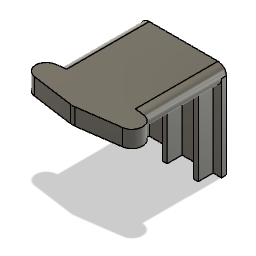
ServoBarMount (Autodesk Fusion 360 design; units mm, degrees)
Autodesk Fusion 360 part; units mm, degrees
sketch "Sketch1" plane through (0, 0, 0) normal (0, 1, 0) x (1, 0, 0)
  line L0 (0, 0) -> (16.3, 0) construction
  line L1 (2.9047, 2.75) -> (2.9047, -2.75) construction
  line L2 (2.9047, 2.75) -> (14.4306, 1.9957)
  line L3 (2.9047, -2.75) -> (14.4306, -1.9957)
  line L4 (0, 4) -> (0, -4) construction
  arc A0 (14.4306, -1.9957) -> (14.4306, 1.9957) centre (14.3, 0) ccw
  line L5 (0.7832, 5.545) -> (14.8035, 3.5646)
  line L6 (0.7832, -5.545) -> (14.8035, -3.5646)
  arc A1 (14.8035, -3.5646) -> (14.8035, 3.5646) centre (14.3, 0) ccw
  line L7 (-2.9047, 2.75) -> (-14.4306, 1.9957)
  line L8 (-0.7832, 5.545) -> (-14.8035, 3.5646)
  line L9 (-2.9047, -2.75) -> (-14.4306, -1.9957)
  line L10 (-0.7832, -5.545) -> (-14.8035, -3.5646)
  arc A2 (-14.4306, 1.9957) -> (-14.4306, -1.9957) centre (-14.3, 0) ccw
  arc A3 (-14.8035, 3.5646) -> (-14.8035, -3.5646) centre (-14.3, 0) ccw
  arc A4 (0.7832, 5.545) -> (-0.7832, 5.545) centre (0, 0) ccw
  arc A5 (-0.7832, -5.545) -> (0.7832, -5.545) centre (0, 0) ccw
  arc A6 (2.9047, 2.75) -> (-2.9047, 2.75) centre (0, 0) ccw
  arc A7 (-2.9047, -2.75) -> (2.9047, -2.75) centre (0, 0) ccw
  line L11 (14.3, 3.6357) -> (14.3, 31.6)
  line L12 (14.3, 30) -> (-14.3, 30)
  line L13 (-14.3, 30) -> (-14.3, 3.6357)
  line L14 (14.3, 31.6) -> (-14.3, 31.6)
  line L15 (-14.3, 31.6) -> (-14.3, 30)
  dimension "d1" = 8
  dimension "d2" = 16.3
  dimension "d3" = 4
  dimension "d5" = 5.5
  dimension "d6" = 1.6
  dimension "d7" = 1.6
  dimension "d8" = 30
  dimension "d16" = 1.6
  constraint coincident L0.start A4.centre
  constraint horizontal L0
  constraint coincident L0 A0.centre
  constraint coincident L0.end A0
  constraint vertical L1
  constraint tangent L2 A0
  constraint tangent L3 A0
  constraint coincident L4.start A6
  constraint coincident L4.end A6
  constraint perpendicular L0 L4
  constraint concentric A0 A1
  constraint concentric A4 A6
  constraint tangent L5 A1
  constraint tangent L5 A4
  constraint tangent L6 A1
  constraint tangent L6 A4
  constraint symmetric L1.start L4 L7.start
  constraint symmetric L1.end L4 L9.start
  constraint symmetric L2.end L4 L7.end
  constraint symmetric L3.end L4 L9.end
  constraint symmetric L4 A0 A2
  constraint symmetric L4 L5.start L8.start
  constraint symmetric L4 L5.end L8.end
  constraint symmetric L4 L6.start L10.start
  constraint symmetric L4 L6.end L10.end
  constraint symmetric L4 A1 A3
  constraint coincident L9.start A6
  constraint concentric A4 A5
  constraint tangent L10 A5
  constraint concentric A6 A7
  constraint vertical L11
  constraint horizontal L12
  constraint vertical L13
  constraint coincident L8 L13.end
  constraint vertical A0.centre L11.start
  constraint vertical A2.centre L13.end
  constraint coincident L5 L11.start
  constraint horizontal L14
  constraint vertical L15
  constraint coincident L11.end L14.start
  constraint coincident L12.start L11
  measures "d1" diameter of A6
  measures "d2" distance of L0.start L0.end
  measures "d3" diameter of A0
  measures "d5" distance of L1.start L1.end
  measures "d6" distance of A0 A1
  measures "d7" distance of A4 A6
  measures "d8" distance of L0.start L12
  measures "d16" distance of L12.end L14.end
extrude "Extrude1" add sketch "Sketch1" along normal blind 1.6 contours L2 L3 A0 L7 L9 A2 A6 A7 | L5 L8 A4 L11 L12 L13 | L5 L6 A1 L8 L10 A3 A4 A5 | L11 L12 L14 L15
extrude "Extrude2" add sketch "Sketch1" against normal blind 4 contours L5 L8 A4 L11 L12 L13 | L5 L6 A1 L8 L10 A3 A4 A5
extrude "Extrude3" add sketch "Sketch1" against normal blind 30 contours L11 L12 L14 L15
fillet "Fillet1" radius 2.8 4 edges at (14.3, 1.6, -17.6179) (14.3, -4, -16.8179) (-14.3, 1.6, -17.6179) (-14.3, -4, -16.8179)
ref_plane "WorkPlane1" through (0.3, -15.6, -30.8) normal (1, 0, 0) x (0, 0, -1)
ref_plane "WorkPlane2" through (-11.5, -15.6, -30.8) normal (-1, 0, 0) x (0, 0, 1)
ref_plane "WorkPlane3" through (11.5, -15.6, -30.8) normal (1, 0, 0) x (0, 0, -1)
sketch "Sketch2" plane through (0.3, -15.6, -30.8) normal (1, 0, 0) x (0, 0, -1)
  line L0 (-0.8, 14.4) -> (-0.8, -14.4)
  line L1 (-0.8, -14.4) -> (-5.8, -14.4)
  line L2 (-5.8, -14.4) -> (-5.8, 11.6)
  line L3 (-5.8, 11.6) -> (-0.8, 11.6)
  line L4 (-0.8, 11.6) -> (-0.8, -14.4)
  line L5 (-26.7688, 11.6) -> (-0.8, 11.6)
  dimension "d25" = 5
  constraint horizontal L1
  constraint vertical L2
  constraint horizontal L3
  constraint vertical L4
  constraint coincident L0.end L1.start
  constraint collinear L3 L5
  measures "d25" distance of L0.end L1.end
sketch "Sketch3" plane through (-11.5, -15.6, -30.8) normal (-1, 0, 0) x (0, 0, -1)
  line L0 (-5.8, 14.4) -> (-5.8, -11.6)
  line L1 (-0.8, 14.4) -> (-5.8, 14.4)
  line L2 (-0.8, -11.6) -> (-0.8, 14.4)
  line L3 (-5.8, -11.6) -> (-0.8, -11.6)
sketch "Sketch4" plane through (11.5, -15.6, -30.8) normal (1, 0, 0) x (0, 0, -1)
  line L0 (-5.8, -14.4) -> (-5.8, 11.6)
  line L1 (-0.8, -14.4) -> (-5.8, -14.4)
  line L2 (-0.8, 11.6) -> (-0.8, -14.4)
  line L3 (-5.8, 11.6) -> (-0.8, 11.6)
extrude "Extrude4" add sketch "Sketch2" along normal mid plane 1.6
extrude "Extrude5" add sketch "Sketch4" against normal blind 1.6
extrude "Extrude6" add sketch "Sketch3" against normal blind 1.6
equation "d7 = d6"
